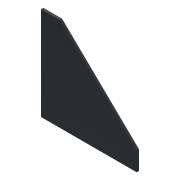
# Autodesk Inventor part: brak1
Saved by Autodesk Inventor 2015 (Build 190159000, 159)
## iProperties
Created: 2015-03-14
Part Number: brak1
Material: Iron, Gray
Document SubType Name: Modeling
Designer: Jaden
Density: 7.15 g/cm^3
Appearance: Iron Gray
Author: Jaden
Autodesk Inventor part; units mm, degrees
ref_plane "YZ Plane" through (0, 0, 0) normal (1, 0, 0) x (0, 1, 0)
ref_plane "XZ Plane" through (0, 0, 0) normal (0, 1, 0) x (-1, 0, 0)
ref_plane "XY Plane" through (0, 0, 0) normal (0, 0, 1) x (1, 0, 0)
sketch "Sketch1" plane through (0, 0, 0) normal (0, 0, 1) x (1, 0, 0)
  line L0 (0, 0) -> (0, 127)
  line L1 (0, 0) -> (130.175, 0)
  line L2 (130.175, 0) -> (130.175, 25.4)
  line L3 (0, 127) -> (25.4, 127)
  line L4 (25.4, 127) -> (130.175, 25.4)
  dimension "d1" = 127
  dimension "d10" = 130.175
  dimension "d11" = 25.4
  dimension "d14" = 25.4
  constraints: 10 end point, 2 horizontal, 1 perpendicular, 1 vertical
  measures "d1" distance of L0.start L0.end
  measures "d10" distance of L0.start L1.end
  measures "d11" distance of L1.end L2.end
  measures "d14" distance of L0.end L3.end
extrude "Extrusion4" add sketch "Sketch1" along normal blind 3.175
body "Solid4"
